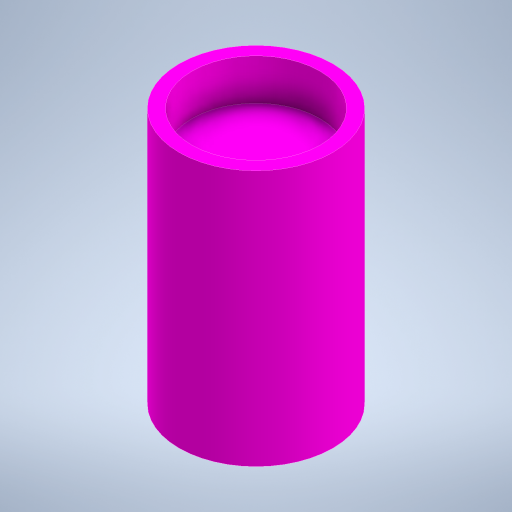
# Autodesk Inventor part: магнит_стойка
Saved by Autodesk Inventor 2023 (Build 270158000, 158)
## iProperties
Created: 2025-02-04
Part Number: магнит_стойка
Material: Типовые
Document SubType Name: Modeling
Designer: baranovaem
Density: 1 g/cm^3
Appearance: Пурпурный
Author: baranovaem
Autodesk Inventor part; units mm, degrees
ref_plane "YZ Plane" through (0, 0, 0) normal (1, 0, 0) x (0, 1, 0)
ref_plane "XZ Plane" through (0, 0, 0) normal (0, 1, 0) x (-1, 0, 0)
ref_plane "XY Plane" through (0, 0, 0) normal (0, 0, 1) x (1, 0, 0)
sketch "Эскиз1" plane through (0, 0, 0) normal (0, 1, 0) x (-1, 0, 0)
  circle A0 centre (0, 0) radius 15
  circle A1 centre (0, 0) radius 12.5
  dimension "d0" = 30
  dimension "d1" = 25
  constraints: 2 centre point, 2 coincident
  measures "d0" diameter of A0
  measures "d1" diameter of A1
extrude "Выдавливание1" add sketch "Эскиз1" along normal blind 50
sketch "Эскиз2" plane through (0, 0, 0) normal (0, -1, 0) x (1, 0, 0)
  circle A0 centre (0, 0) radius 15 projected
extrude "Выдавливание2" add sketch "Эскиз2" against normal blind 42
